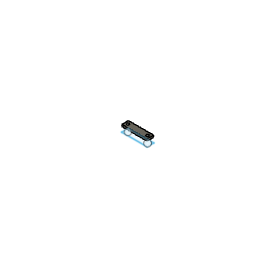
Power Switch Retainer (Autodesk Fusion 360 design; units mm, degrees)
Autodesk Fusion 360 part; units mm, degrees
sketch "sketch 297" plane through (0, 0, 7.7091) normal (0, 0, -1) x (1, 0, 0)
  circle A0 centre (8.05, 57.0409) radius 1.125
  circle A1 centre (-8.35, 57.0409) radius 1.125
  line L0 (-10.7, 59.8409) -> (-10.7, 54.3409)
  line L1 (10.4, 54.3409) -> (-10.7, 54.3409)
  line L2 (10.4, 54.3409) -> (10.4, 59.8409)
  line L3 (-10.7, 59.8409) -> (10.4, 59.8409)
extrude "Extrude1" add sketch "sketch 297" against normal blind 1.6 from surface at -4.05
